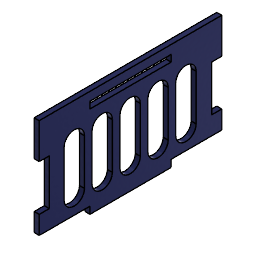
front_wall (Autodesk Fusion 360 design; units mm, degrees)
part number: 2026-06-29-22-34-53-178
Autodesk Fusion 360 part; units mm, degrees
sketch "Sketch1" plane through (0, 0, 0) normal (1, 0, 0) x (0, 1, 0)
  line L0 (0, 0) -> (180, 0)
  line L1 (180, 0) -> (180, 25)
  line L2 (180, 25) -> (170, 25)
  line L3 (170, 25) -> (170, 70)
  line L4 (170, 70) -> (180, 70)
  line L5 (180, 70) -> (180, 105)
  line L6 (180, 105) -> (170, 105)
  line L7 (170, 105) -> (0, 105)
  line L8 (0, 105) -> (0, 70)
  line L9 (0, 70) -> (10, 70)
  line L10 (10, 70) -> (10, 25)
  line L11 (10, 25) -> (0, 25)
  line L12 (0, 25) -> (0, 0)
  line L13 (0, 0) -> (50, 0)
  line L14 (50, 0) -> (50, 7)
  line L15 (50, 7) -> (0, 7)
  line L16 (0, 7) -> (0, 0)
  line L17 (180, 0) -> (130, 0)
  line L18 (130, 0) -> (130, 7)
  line L19 (130, 7) -> (180, 7)
  line L20 (180, 7) -> (180, 0)
  dimension "d1" = 180
  dimension "d2" = 10
  dimension "d4" = 25
  dimension "d5" = 105
  dimension "d6" = 10
  dimension "d20" = 35
  dimension "d22" = 7
  dimension "d23" = 50
  dimension "d26" = 80
  constraint coincident L0.start L12.end
  constraint horizontal L0
  constraint perpendicular L0 L1
  constraint perpendicular L1 L2
  constraint perpendicular L2 L3
  constraint perpendicular L3 L4
  constraint perpendicular L4 L5
  constraint perpendicular L5 L6
  constraint perpendicular L5 L7
  constraint perpendicular L4 L8
  constraint perpendicular L8 L9
  constraint perpendicular L4 L10
  constraint perpendicular L10 L11
  constraint perpendicular L0 L12
  constraint collinear L1 L5
  constraint collinear L8 L12
  constraint collinear L2 L11
  constraint collinear L4 L9
  constraint horizontal L13
  constraint vertical L14
  constraint horizontal L15
  constraint vertical L16
  constraint horizontal L17
  constraint vertical L18
  constraint horizontal L19
  constraint vertical L20
  constraint equal L15 L19
  constraint equal L14 L18
  measures "d1" distance of L0.start L0.end
  measures "d2" distance of L10.end L11.end
  measures "d4" distance of L11.end L0.start
  measures "d5" distance of L0 L7
  measures "d6" distance of L1.end L2.end
  measures "d20" distance of L7.end L8.end
  measures "d22" distance of L13.end L14.end
  measures "d23" distance of L14.end L15.end
  measures "d26" distance of L14 L18
extrude "Extrude1" add sketch "Sketch1" along normal blind 5
sketch "Sketch2" plane through (5, 0, 0) normal (1, 0, 0) x (0, 1, 0)
  line L0 (0, 25) -> (0, 0)
  line L1 (0, 0) -> (180, 0)
  line L2 (180, 0) -> (180, 25)
  line L3 (180, 25) -> (170, 25)
  line L4 (170, 25) -> (170, 70)
  line L5 (170, 70) -> (180, 70)
  line L6 (180, 70) -> (180, 105)
  line L7 (180, 105) -> (0, 105)
  line L8 (0, 105) -> (0, 70)
  line L9 (0, 70) -> (10, 70)
  line L10 (10, 70) -> (10, 25)
  line L11 (10, 25) -> (0, 25)
  line L12 (134.6138, 69.8664) -> (134.6138, 24.8664)
  arc A0 (134.6138, 24.8664) -> (154.6138, 24.8664) centre (144.6138, 24.8664) ccw
  line L13 (154.6138, 24.8664) -> (154.6138, 69.8664)
  arc A1 (154.6138, 69.8664) -> (134.6138, 69.8664) centre (144.6138, 69.8664) ccw
  line L14 (144.6138, 69.8664) -> (144.6138, 24.8664) construction
  line L15 (50, 96.5) -> (130, 96.5)
  line L16 (130, 96.5) -> (130, 90)
  line L17 (130, 90) -> (50, 90)
  line L18 (50, 90) -> (50, 96.5)
  dimension "d9" = 20
  dimension "d15" = 90
  dimension "d16" = 6.5
  dimension "d17" = 80
  dimension "d18" = 50
  dimension "d25" = 45
  constraint tangent L12 A0
  constraint tangent A0 L13
  constraint parallel L12 L13
  constraint tangent L13 A1
  constraint tangent L12 A1
  constraint horizontal L15
  constraint vertical L16
  constraint horizontal L17
  constraint vertical L18
  measures "d9" diameter of A0
  measures "d15" distance of L1 L17
  measures "d16" distance of L15 L17
  measures "d17" distance of L16.end L17.end
  measures "d18" distance of L6 L16
  measures "d25" distance of A0.end L13.end
extrude "Extrude2" cut sketch "Sketch2" against normal through all contours L12 A0 L13 A1
pattern_linear "R-Pattern1" count 1 spacing 0 along (0, 0, -1) count 5 spacing 27.5 along (0, -1, 0) of "Extrude2"
extrude "Extrude3" cut sketch "Sketch2" against normal through all contours L15 L16 L17 L18
extrude "Extrude4" cut sketch "Sketch1" along normal through all contours L0 L12 L13 L14 L15 L16 | L0 L1 L17 L18 L19 L20
